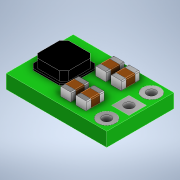
# Autodesk Inventor part: S9V11F5
Saved by Autodesk Inventor 2021 (Build 250183000, 183)
## iProperties
Created: 2021-07-23
Part Number: S9V11F5
Material: Generic
Document SubType Name: Modeling
Designer: ermoz
Density: 1 g/cm^3
Appearance: Default
Author: ermoz
Autodesk Inventor part; units mm, degrees
ref_plane "YZ Plane" through (0, 0, 0) normal (1, 0, 0) x (0, 1, 0)
ref_plane "XZ Plane" through (0, 0, 0) normal (0, 1, 0) x (-1, 0, 0)
ref_plane "XY Plane" through (0, 0, 0) normal (0, 0, 1) x (1, 0, 0)
sketch "Sketch1" plane through (0, 0, 0) normal (0, 1, 0) x (-1, 0, 0)
  line L0 (-5.715, 3.81) -> (5.715, 3.81)
  line L1 (5.715, 3.81) -> (5.715, -3.81)
  line L2 (5.715, -3.81) -> (-5.715, -3.81)
  line L3 (-5.715, -3.81) -> (-5.715, 3.81)
  line L4 (-5.715, 3.81) -> (5.715, -3.81) construction
  line L5 (5.715, 3.81) -> (-5.715, -3.81) construction
  point P0 (0, 0)
  dimension "d0" = 11.43
  dimension "d1" = 7.62
  constraints: 12 end point, 2 midpoint, 2 parallel, 1 horizontal, 1 perpendicular
  measures "d0" distance of L1.end L2.end
  measures "d1" distance of L0.end L1.end
extrude "Extrusion1" add sketch "Sketch1" along normal blind 1.6
sketch "Sketch2" plane through (0, 1.6, 0) normal (0, 1, 0) x (1, 0, 0)
  circle A0 centre (4.4345, 0) radius 0.5
  circle A1 centre (4.4345, 2.54) radius 0.5
  circle A2 centre (4.4345, 2.54) radius 1
  line L0 (3.4345, 1) -> (5.4345, 1)
  line L1 (5.4345, 1) -> (5.4345, -1)
  line L2 (5.4345, -1) -> (3.4345, -1)
  line L3 (3.4345, -1) -> (3.4345, 1)
  line L4 (3.4345, 1) -> (5.4345, -1) construction
  line L5 (5.4345, 1) -> (3.4345, -1) construction
  line L6 (5.4345, 1) -> (5.4345, 2.54) construction
  line L7 (3.4345, 1) -> (3.4345, 2.54) construction
  line L8 (0, 0) -> (0.9361, 0) construction
  circle A3 centre (4.4345, -2.54) radius 0.5
  circle A4 centre (4.4345, -2.54) radius 1
  line L9 (5.4345, 2.54) -> (5.715, 2.54)
  line L10 (5.715, -3.81) -> (5.715, 3.81) projected
  line L11 (4.2897, 3.5295) -> (4.2897, 3.81)
  line L12 (5.715, 3.81) -> (-5.715, 3.81) projected
  point P0 (5.4345, -2.54)
  point P1 (3.4345, -2.54)
  point P2 (4.4345, 0)
  dimension "d4" = 2.54
  dimension "d5" = 1
  dimension "d6" = 2
  constraints: 22 end point, 5 centre point, 5 point on circle, 4 symmetric about line, 3 horizontal, 3 midpoint, 3 perpendicular, 3 point on line, 2 coincident, 2 collinear, 2 parallel, 2 tangent, 1 equal radius, 1 vertical, 1 vertical alignment, 2 other
  measures "d4" distance of A0.centre A1.centre
  measures "d5" diameter of A1
  measures "d6" diameter of A2
extrude "Extrusion2" cut sketch "Sketch2" against normal through all contours A0 | A1 | A2 | L0 L1 L2 L3 | A3 | A4
extrude "Extrusion3" add sketch "Sketch2" against normal up to surface (1.6 mm away) separate body contours A2 | L0 L1 L2 L3 | A4
sketch "Sketch3" plane through (0, 1.6, 0) normal (0, 1, 0) x (1, 0, 0)
  line L0 (-4.965, -2) -> (-0.965, -2)
  line L1 (-0.965, -2) -> (-0.965, 2)
  line L2 (-0.965, 2) -> (-4.965, 2)
  line L3 (-4.965, 2) -> (-4.965, -2)
  line L4 (-4.965, -2) -> (-0.965, 2) construction
  line L5 (-0.965, -2) -> (-4.965, 2) construction
  line L6 (0, 0) -> (1.5246, 0)
  line L7 (-0.3715, -1) -> (0.8785, -1)
  line L8 (0.8785, -1) -> (0.8785, -1.5)
  line L9 (0.8785, -1.5) -> (-0.3715, -1.5)
  line L10 (-0.3715, -1.5) -> (-0.3715, -1)
  line L11 (-0.3715, -1.5) -> (0.8785, -1.5)
  line L12 (0.8785, -1.5) -> (0.8785, -2.5)
  line L13 (0.8785, -2.5) -> (-0.3715, -2.5)
  line L14 (-0.3715, -2.5) -> (-0.3715, -1.5)
  line L15 (-0.3715, -2.5) -> (0.8785, -2.5)
  line L16 (0.8785, -2.5) -> (0.8785, -3)
  line L17 (0.8785, -3) -> (-0.3715, -3)
  line L18 (-0.3715, -3) -> (-0.3715, -2.5)
  line L19 (1.3785, -1) -> (2.6285, -1)
  line L20 (2.6285, -1) -> (2.6285, -1.5)
  line L21 (2.6285, -1.5) -> (1.3785, -1.5)
  line L22 (1.3785, -1.5) -> (1.3785, -1)
  line L23 (1.3785, -1.5) -> (2.6285, -1.5)
  line L24 (2.6285, -1.5) -> (2.6285, -2.5)
  line L25 (2.6285, -2.5) -> (1.3785, -2.5)
  line L26 (1.3785, -2.5) -> (1.3785, -1.5)
  line L27 (1.3785, -2.5) -> (2.6285, -2.5)
  line L28 (2.6285, -2.5) -> (2.6285, -3)
  line L29 (2.6285, -3) -> (1.3785, -3)
  line L30 (1.3785, -3) -> (1.3785, -2.5)
  line L31 (-0.3715, 1) -> (0.8785, 1)
  line L32 (0.8785, 1) -> (0.8785, 1.5)
  line L33 (0.8785, 1.5) -> (-0.3715, 1.5)
  line L34 (-0.3715, 1.5) -> (-0.3715, 1)
  line L35 (-0.3715, 1.5) -> (0.8785, 1.5)
  line L36 (0.8785, 1.5) -> (0.8785, 2.5)
  line L37 (0.8785, 2.5) -> (-0.3715, 2.5)
  line L38 (-0.3715, 2.5) -> (-0.3715, 1.5)
  line L39 (-0.3715, 2.5) -> (0.8785, 2.5)
  line L40 (0.8785, 2.5) -> (0.8785, 3)
  line L41 (0.8785, 3) -> (-0.3715, 3)
  line L42 (-0.3715, 3) -> (-0.3715, 2.5)
  line L43 (1.3785, 1) -> (2.6285, 1)
  line L44 (2.6285, 1) -> (2.6285, 1.5)
  line L45 (2.6285, 1.5) -> (1.3785, 1.5)
  line L46 (1.3785, 1.5) -> (1.3785, 1)
  line L47 (1.3785, 1.5) -> (2.6285, 1.5)
  line L48 (2.6285, 1.5) -> (2.6285, 2.5)
  line L49 (2.6285, 2.5) -> (1.3785, 2.5)
  line L50 (1.3785, 2.5) -> (1.3785, 1.5)
  line L51 (1.3785, 2.5) -> (2.6285, 2.5)
  line L52 (2.6285, 2.5) -> (2.6285, 3)
  line L53 (2.6285, 3) -> (1.3785, 3)
  line L54 (1.3785, 3) -> (1.3785, 2.5)
  point P0 (-2.965, 0)
  point P1 (-2.965, 0)
  point P2 (0.8785, 1.5)
  dimension "d11" = 4
  dimension "d16" = 2
  dimension "d17" = 1.25
  dimension "d18" = 0.5
  dimension "d19" = 0.5
  dimension "d20" = 1
  constraints: 110 end point, 20 symmetric about line, 14 parallel, 9 point on line, 8 horizontal, 7 perpendicular, 4 collinear, 3 equal length, 3 midpoint
  measures "d11" distance of L2.end L0.start
  measures "d16" distance between parallel lines of L17 L7
  measures "d17" distance of L16.end L17.end
  measures "d18" distance of L17.end L13.end
  measures "d19" distance between parallel lines of L30 L16
  measures "d20" distance between parallel lines of L6 L7
extrude "Extrusion4" add sketch "Sketch3" along normal blind 1.2 separate body contours L3 L2 L1 L0
extrude "Extrusion5" add sketch "Sketch3" along normal blind 1 separate body contours L7 L8 L9 L10 | L13 L16 L17 L18 | L19 L20 L21 L22 | L25 L28 L29 L30 | L34 L33 L32 L31 | L42 L41 L40 L37 | L46 L45 L44 L43 | L54 L53 L52 L49
extrude "Extrusion6" add sketch "Sketch3" along normal up to surface (1 mm away) separate body contours L9 L12 L13 L14 | L21 L24 L25 L26 | L38 L37 L36 L33 | L50 L49 L48 L45
fillet "Fillet1" radius 0.1 46 edges at (2.6285, 2.6, 1.25) (2.6285, 2.6, 2.75) (2.6285, 1.6, 2.75) (2.6285, 1.6, 1.25) (1.3785, 1.6, 1.25) (1.3785, 1.6, 2.75) (1.3785, 2.6, 2.75) (1.3785, 2.6, 1.25) (2.6285, 1.6, -1.25) (2.6285, 1.6, -2.75) (2.6285, 2.6, -2.75) (2.6285, 2.6, -1.25) (1.3785, 1.6, -2.75) (1.3785, 1.6, -1.25) (1.3785, 2.6, -1.25) (1.3785, 2.6, -2.75) (-0.3715, 1.6, -2.75) (-0.3715, 1.6, -1.25) (-0.3715, 2.6, -1.25) (-0.3715, 2.6, -2.75) (0.8785, 2.6, -1.25) (0.8785, 1.6, -1.25) (0.8785, 1.6, -2.75) (0.8785, 2.6, 2.75) (0.8785, 2.6, 1.25) (0.8785, 1.6, 2.75) (0.8785, 1.6, 1.25) (-0.3715, 1.6, 1.25) (-0.3715, 1.6, 2.75) (-0.3715, 2.6, 2.75) (-0.3715, 2.6, 1.25) (2.6285, 2.6, 2) (2.6285, 1.6, 2) (1.3785, 1.6, 2) (1.3785, 2.6, 2) (2.6285, 1.6, -2) (2.6285, 2.6, -2) (1.3785, 1.6, -2) (1.3785, 2.6, -2) (-0.3715, 1.6, -2) (-0.3715, 2.6, -2) (0.8785, 1.6, -2) (0.8785, 2.6, 2) (0.8785, 1.6, 2) (-0.3715, 1.6, 2) (-0.3715, 2.6, 2)
sketch "Sketch4" plane through (0, 2.8, 0) normal (0, 1, 0) x (1, 0, 0)
  line L0 (-0.965, 2) -> (-4.965, 2) projected
  line L1 (-0.965, -2) -> (-0.965, 2) projected
  line L2 (-0.965, 2) -> (-4.965, 2) projected
  line L3 (-4.965, 2) -> (-4.965, -2) projected
  line L4 (-4.965, -2) -> (-0.965, -2) projected
  line L5 (-4.715, -1.75) -> (-4.715, 1.75)
  line L6 (-4.715, 1.75) -> (-1.215, 1.75)
  line L7 (-1.215, 1.75) -> (-1.215, -1.75)
  line L8 (-1.215, -1.75) -> (-4.715, -1.75)
  point P0 (0, 0)
  dimension "d28" = 0.25
  constraints: 8 end point, 3 other
  measures "d28" distance between parallel lines of L3 L5
extrude "Extrusion7" cut sketch "Sketch4" against normal blind 1 bodies 3
chamfer "Chamfer1" distance 0.5 angle 45 8 edges at (-1.215, 2.3, 1.75) (-0.965, 1.7, 2) (-4.965, 1.7, 2) (-4.715, 2.3, 1.75) (-4.965, 1.7, -2) (-4.715, 2.3, -1.75) (-1.215, 2.3, -1.75) (-0.965, 1.7, -2)
sketch "Sketch5" plane through (0, 0, 0) normal (0, -1, 0) x (1, 0, 0)
  line L0 (-1.9712, -1.375) -> (-3.9712, -1.375)
  line L1 (-3.9712, -1.375) -> (-3.9712, 1.375)
  line L2 (-3.9712, 1.375) -> (-1.9712, 1.375)
  line L3 (-1.9712, 1.375) -> (-1.9712, -1.375)
  line L4 (-1.9712, -1.375) -> (-3.9712, 1.375) construction
  line L5 (-3.9712, -1.375) -> (-1.9712, 1.375) construction
  line L6 (0, 0) -> (-0.8421, 0)
  point P0 (-2.9712, 0)
  point P1 (-2.9712, 0)
  dimension "d34" = 2
  dimension "d35" = 2.75
  constraints: 14 end point, 3 midpoint, 2 horizontal, 2 parallel, 1 perpendicular, 1 point on line
  measures "d34" distance of L1.end L2.end
  measures "d35" distance of L0.end L1.end
extrude "Extrusion8" add sketch "Sketch5" along normal blind 1 separate body
body "Solid1"
body "Solid2"
body "Solid3"
body "Solid4"
body "Solid5"
body "Solid6"
